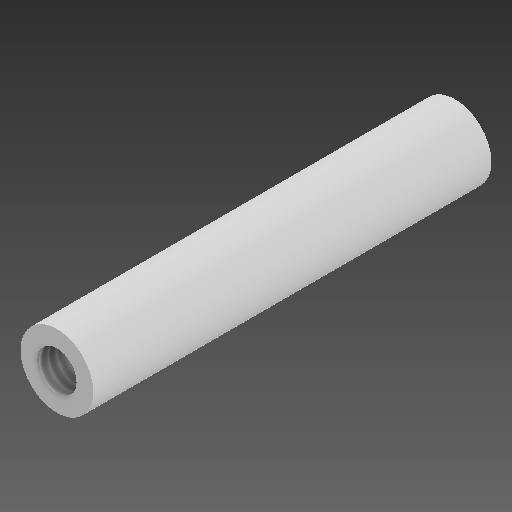
# Autodesk Inventor part: GEARBOX STANDOFFS
Saved by Autodesk Inventor 2020 (Build 240168000, 168)
## iProperties
Created: 2021-01-18
Part Number: GEARBOX STANDOFFS
Material: Generic
Document SubType Name: Modeling
Designer: lucky
Density: 1 g/cm^3
Appearance: Default
Mass: 0.76369 g
Surface Area: 8.79442 cm^2
Volume: 0.76369 cm^3
Author: lucky
Autodesk Inventor part; units mm, degrees
ref_plane "YZ Plane" through (0, 0, 0) normal (1, 0, 0) x (0, 1, 0)
sketch "Sketch2" plane through (0, 0, 0) normal (0, 0, 1) x (1, 0, 0)
  circle A0 centre (0, 0) radius 3
  dimension "d0" = 6
  constraints: 1 centre point, 1 coincident
  measures "d0" diameter of A0
ref_plane "Work Plane1" through (-3.0381, -3.0381, 30.2492) normal (0, 0, -1) x (0, 1, 0)
ref_plane "Work Plane2" through (-3.0898, -3.0898, 32.8492) normal (0, 0, -1) x (0.0301, 0.9995, 0)
extrude "Extrusion1" add sketch "Sketch2" along normal up to surface (32.8492 mm away)
sketch "Sketch3" plane through (0, 0, 32.8492) normal (0, 0, 1) x (1, 0, 0)
  point P0 (0, 0)
  point P1 (0, 0)
  constraints: 1 coincident
hole "Hole1" at (0, 0, 32.8492) direction (0, 0, -1) diameter 3.242 depth 10 thread size "M4x0.7" class "6H" standard "ISO Metric profile"
sketch "Sketch4" plane through (0, 0, 0) normal (0, 0, -1) x (-1, 0, 0)
  circle A0 centre (0, 0) radius 1.621 projected
  point P0 (0, 0)
  constraints: 1 coincident
hole "Hole2" at (0, 0, 0) direction (0, 0, 1) diameter 3.242 depth 10 thread size "M4x0.7" class "6H" standard "ISO Metric profile"
body "Solid1"
